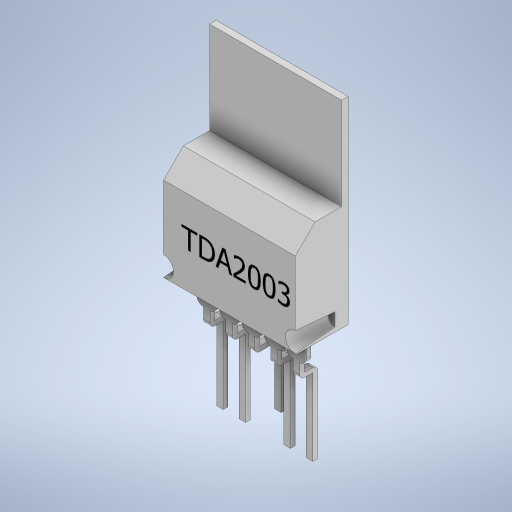
# Autodesk Inventor part: TDA2003
Saved by Autodesk Inventor 2024 (Build 280153000, 153)
## iProperties
Created: 2023-12-15
Part Number: TDA2003
Material: Generic
Document SubType Name: Sheet Metal
Designer: user
Density: 1 g/cm^3
Sheet Metal Rule: Default
Appearance: Default
Author: user
Autodesk Inventor part; units mm, degrees
sketch "Sketch1" plane through (0, 0, 0) normal (0, 0, 1) x (1, 0, 0)
  line L0 (0, 0) -> (10, 0)
  line L1 (10, 0) -> (10, 5)
  line L2 (10, 5) -> (0, 5)
  line L3 (0, 5) -> (0, 0)
  line L4 (0, 0) -> (0, 1.6)
  line L5 (0, 0) -> (0, 0.1)
  arc A0 (0, 0.1) -> (0, 1.6) centre (0, 0.85) ccw
  line L6 (10, 0) -> (10, 1.6)
  line L7 (10, 0) -> (10, 0.1)
  arc A1 (10, 1.6) -> (10, 0.1) centre (10, 0.85) ccw
  dimension "d0" = 10
  dimension "d1" = 5
  dimension "d2" = 1.6
  dimension "d3" = 0.1
  dimension "d4" = 0.75
  dimension "d5" = 1.6
  dimension "d6" = 0.1
  dimension "d7" = 0.75
  constraints: 16 end point, 4 point on circle, 4 point on line, 2 centre point, 2 parallel, 1 horizontal, 1 perpendicular
  measures "d0" distance of L2.end L1.end
  measures "d1" distance of L1.end L0.end
  measures "d2" distance of L0.start L4.end
  measures "d3" distance of L0.start L5.end
  measures "d4" radius of A0
  measures "d5" distance of L0.end L6.end
  measures "d6" distance of L0.end L7.end
  measures "d7" radius of A1
extrude "Extrusion1" add sketch "Sketch1" along normal blind 1 contours L3 A0 | A1 L1
extrude "Extrusion2" add sketch "Sketch1" along normal blind 4 contours L3 A0 L2 L1 A1 L0
draft "FaceDraft1" angle 5 pull direction (0, 0, 1) faces at (9.8797, 0.1097, 2) fixed edges at (9.25, 0.85, 4)
draft "FaceDraft2" angle 5 pull direction (0, 0, 1) faces at (0.0603, 0.1024, 3) fixed edges at (0.75, 0.85, 4)
sketch "Sketch2" plane through (0, 5, 0) normal (0, 1, 0) x (1, 0, 0)
  line L0 (0, -1) -> (0, -4) projected
  line L1 (10, 0) -> (0, 0) projected
  line L2 (0, -4) -> (10, -4)
  line L3 (10, -4) -> (10, 0)
  line L4 (10, 0) -> (0, 0)
  line L5 (0, 0) -> (0, -4)
  line L6 (0, 0) -> (10, 0)
  line L7 (10, 0) -> (10, -0.5)
  line L8 (10, -0.5) -> (0, -0.5)
  line L9 (0, -0.5) -> (0, 0)
  dimension "d14" = 0.5
  constraints: 16 end point, 4 parallel, 2 horizontal, 2 perpendicular, 1 point on line
  measures "d14" distance of L6.end L7.end
extrude "Extrusion3" add sketch "Sketch2" along normal blind 3
sketch "Sketch3" plane through (0, 8, 0) normal (0, 1, 0) x (1, 0, 0)
  line L0 (10, 0) -> (10, -4) projected
  line L1 (0, 0) -> (10, 0)
  line L2 (10, 0) -> (10, -0.5)
  line L3 (10, -0.5) -> (0, -0.5)
  line L4 (0, -0.5) -> (0, 0)
  dimension "d17" = 0.5
  constraints: 8 end point, 2 parallel, 1 horizontal, 1 perpendicular, 1 point on line
  measures "d17" distance of L1.end L2.end
extrude "Extrusion4" add sketch "Sketch3" along normal blind 7
chamfer "Chamfer1" distance 1.5 angle 45 1 edges at (5, 8, 4)
chamfer "Chamfer2" distance 0.1 angle 45 1 edges at (5, 0, 4)
sketch "Sketch4" plane through (0, 0, 0) normal (0, -1, 0) x (1, 0, 0)
  line L0 (0.75, 1.9689) -> (2.45, 1.9689)
  line L1 (2.45, 1.9689) -> (4.15, 1.9689)
  line L2 (4.15, 1.9689) -> (5.85, 1.9689)
  line L3 (5.85, 1.9689) -> (7.55, 1.9689)
  line L4 (7.55, 1.9689) -> (9.25, 1.9689)
  line L5 (10, 0) -> (10, 3.9) projected
  line L6 (0, 3.9) -> (10, 3.9) projected
  line L7 (3.3, 1.9689) -> (3.3, 3.9)
  line L8 (5, 1.9689) -> (5, 3.9)
  line L9 (6.7, 1.9689) -> (6.7, 3.9)
  line L10 (8.4, 1.9689) -> (8.4, 3.9)
  line L11 (0.75, 1.9689) -> (0.85, 1.9689)
  line L12 (2.45, 1.9689) -> (2.55, 1.9689)
  line L13 (4.15, 1.9689) -> (4.25, 1.9689)
  line L14 (5.85, 1.9689) -> (5.95, 1.9689)
  line L15 (7.55, 1.9689) -> (7.65, 1.9689)
  line L16 (0.85, 1.9689) -> (2.35, 1.9689)
  line L17 (2.35, 1.9689) -> (2.35, 2.3189)
  line L18 (2.35, 2.3189) -> (0.85, 2.3189)
  line L19 (0.85, 2.3189) -> (0.85, 1.9689)
  line L20 (2.55, 1.9689) -> (4.05, 1.9689)
  line L21 (4.05, 1.9689) -> (4.05, 2.3189)
  line L22 (4.05, 2.3189) -> (2.55, 2.3189)
  line L23 (2.55, 2.3189) -> (2.55, 1.9689)
  line L24 (4.25, 1.9689) -> (5.75, 1.9689)
  line L25 (5.75, 1.9689) -> (5.75, 2.3189)
  line L26 (5.75, 2.3189) -> (4.25, 2.3189)
  line L27 (4.25, 2.3189) -> (4.25, 1.9689)
  line L28 (5.95, 1.9689) -> (7.45, 1.9689)
  line L29 (7.45, 1.9689) -> (7.45, 2.3189)
  line L30 (7.45, 2.3189) -> (5.95, 2.3189)
  line L31 (5.95, 2.3189) -> (5.95, 1.9689)
  line L32 (7.65, 1.9689) -> (9.15, 1.9689)
  line L33 (9.15, 1.9689) -> (9.15, 2.3189)
  line L34 (9.15, 2.3189) -> (7.65, 2.3189)
  line L35 (7.65, 2.3189) -> (7.65, 1.9689)
  line L36 (1.6, 1.9689) -> (1.6, 3.9)
  point P0 (0, 0)
  dimension "d27" = 1.7
  dimension "d28" = 1.7
  dimension "d29" = 1.7
  dimension "d30" = 1.7
  dimension "d31" = 1.7
  dimension "d32" = 0.1
  dimension "d33" = 0.1
  dimension "d34" = 0.1
  dimension "d35" = 0.1
  dimension "d36" = 0.1
  dimension "d37" = 1.5
  dimension "d38" = 0.35
  dimension "d39" = 1.5
  dimension "d40" = 0.35
  dimension "d41" = 1.5
  dimension "d42" = 0.35
  dimension "d43" = 1.5
  dimension "d44" = 0.35
  dimension "d45" = 1.5
  dimension "d46" = 0.35
  constraints: 70 end point, 13 point on line, 10 parallel, 9 perpendicular, 6 midpoint, 5 horizontal
  measures "d27" distance of L0.start L0.end
  measures "d28" distance of L0.end L1.end
  measures "d29" distance of L1.end L2.end
  measures "d30" distance of L2.end L3.end
  measures "d31" distance of L3.end L4.end
  measures "d32" distance of L0.start L11.end
  measures "d33" distance of L0.end L12.end
  measures "d34" distance of L1.end L13.end
  measures "d35" distance of L2.end L14.end
  measures "d36" distance of L3.end L15.end
  measures "d37" distance of L18.end L17.end
  measures "d38" distance of L17.end L16.end
  measures "d39" distance of L22.end L21.end
  measures "d40" distance of L21.end L20.end
  measures "d41" distance of L26.end L25.end
  measures "d42" distance of L25.end L24.end
  measures "d43" distance of L30.end L29.end
  measures "d44" distance of L29.end L28.end
  measures "d45" distance of L34.end L33.end
  measures "d46" distance of L33.end L32.end
ref_plane "Work Plane2" through (3.3, 0, 1.9689) normal (1, 0, 0) x (0, 0, 1)
ref_plane "Work Plane3" through (5, 0, 1.9689) normal (1, 0, 0) x (0, 0, 1)
ref_plane "Work Plane4" through (6.7, 0, 1.9689) normal (1, 0, 0) x (0, 0, 1)
ref_plane "Work Plane5" through (8.4, 0, 1.9689) normal (1, 0, 0) x (0, 0, 1)
extrude "Extrusion5" add sketch "Sketch4" along normal blind 2 contours L19 L18 L36 L0 | L36 L18 L17 L0 | L23 L22 L7 L1 | L7 L22 L21 L1 | L26 L25 L2 L8 | L8 L2 L27 L26 | L30 L29 L3 L9 | L9 L3 L31 L30 | L34 L33 L4 L10 | L10 L4 L35 L34
fillet "Fillet1" radius 0.5 10 edges at (2.35, -2, 2.1439) (0.85, -2, 2.1439) (2.55, -2, 2.1439) (4.05, -2, 2.1439) (4.25, -2, 2.1439) (5.75, -2, 2.1439) (5.95, -2, 2.1439) (7.45, -2, 2.1439) (7.65, -2, 2.1439) (9.15, -2, 2.1439)
sketch "Sketch5" plane through (8.4, 0, 1.9689) normal (1, 0, 0) x (0, 0, 1)
  line L0 (0.1751, 0) -> (0.1751, 2)
  line L1 (0.1751, 2) -> (0.1751, 2.8)
  line L2 (-0.0249, 3) -> (-0.6249, 3)
  line L3 (-0.8249, 3.2) -> (-0.8249, 9)
  arc A0 (0.1751, 2.8) -> (-0.0249, 3) centre (-0.0249, 2.8) ccw
  arc A1 (-0.8249, 3.2) -> (-0.6249, 3) centre (-0.6249, 3.2) ccw
  point P0 (-1.9689, 0)
  point P1 (1.9311, 0)
  point P2 (0.1751, 3)
  point P3 (-0.8249, 3)
  dimension "d55" = 1.756
  dimension "d56" = 2
  dimension "d57" = 1
  dimension "d58" = 1
  dimension "d59" = 6
  dimension "d60" = 0.2
  constraints: 8 end point, 5 point on line, 4 point on circle, 4 tangent, 2 centre point, 2 perpendicular, 1 equal radius
  measures "d55" distance of point (1.931, 0) L0.start
  measures "d56" distance of L0.start L0.end
  measures "d57" distance of L0.end point (0.175, 3)
  measures "d58" distance of point (0.175, 3) point (-0.825, 3)
  measures "d59" distance of point (-0.825, 3) L3.end
  measures "d60" radius of A0
ref_plane "Work Plane6" through (0, -2, 0) normal (0, -1, 0) x (1, 0, 0)
ref_plane "Work Plane7" through (0, -2, 0) normal (0, -1, 0) x (1, 0, 0)
ref_plane "Work Plane8" through (0, -2, 0) normal (0, -1, 0) x (1, 0, 0)
ref_plane "Work Plane9" through (0, -2, 0) normal (0, -1, 0) x (1, 0, 0)
ref_plane "Work Plane10" through (0, -2, 0) normal (0, -1, 0) x (1, 0, 0)
sketch "Sketch6" plane through (0, -2, 0) normal (0, -1, 0) x (1, 0, 0)
  line L0 (8.65, 2.3189) -> (8.15, 2.3189) projected
  line L1 (8.15, 1.9689) -> (8.65, 1.9689) projected
  line L2 (8.65, 2.3189) -> (8.15, 2.3189)
  line L3 (8.15, 2.3189) -> (8.15, 1.9689)
  line L4 (8.15, 1.9689) -> (8.65, 1.9689)
  line L5 (8.65, 1.9689) -> (8.65, 2.3189)
  point P0 (0, 0)
  constraints: 8 end point, 2 parallel, 1 horizontal, 1 perpendicular
sketch "Sketch7" plane through (6.7, 0, 1.9689) normal (1, 0, 0) x (0, 0, 1)
  line L0 (0.1751, 0) -> (0.1751, 2)
  line L1 (0.1751, 2) -> (0.1751, 2.8)
  line L2 (-0.0249, 3) -> (-0.6249, 3)
  line L3 (-0.8249, 3.2) -> (-0.8249, 9)
  arc A0 (0.1751, 2.8) -> (-0.0249, 3) centre (-0.0249, 2.8) ccw
  arc A1 (-0.8249, 3.2) -> (-0.6249, 3) centre (-0.6249, 3.2) ccw
  point P0 (-1.9689, 0)
  point P1 (1.9311, 0)
  point P2 (0.1751, 3)
  point P3 (-0.8249, 3)
  dimension "d66" = 1.756
  dimension "d67" = 2
  dimension "d68" = 1
  dimension "d69" = 1
  dimension "d70" = 6
  dimension "d71" = 0.2
  constraints: 8 end point, 5 point on line, 4 point on circle, 4 tangent, 2 centre point, 2 perpendicular, 1 equal radius
  measures "d66" distance of point (1.931, 0) L0.start
  measures "d67" distance of L0.start L0.end
  measures "d68" distance of L0.end point (0.175, 3)
  measures "d69" distance of point (0.175, 3) point (-0.825, 3)
  measures "d70" distance of point (-0.825, 3) L3.end
  measures "d71" radius of A0
sketch "Sketch8" plane through (5, 0, 1.9689) normal (1, 0, 0) x (0, 0, 1)
  line L0 (0.1751, 0) -> (0.1751, 2)
  line L1 (0.1751, 2) -> (0.1751, 2.8)
  line L2 (-0.0249, 3) -> (-1.6249, 3)
  line L3 (-1.8249, 3.2) -> (-1.8249, 8)
  arc A0 (0.1751, 2.8) -> (-0.0249, 3) centre (-0.0249, 2.8) ccw
  arc A1 (-1.8249, 3.2) -> (-1.6249, 3) centre (-1.6249, 3.2) ccw
  point P0 (-1.9689, 0)
  point P1 (1.9311, 0)
  point P2 (-0.8249, 3)
  point P3 (0.1751, 3)
  point P4 (-1.8249, 3)
  dimension "d72" = 1.756
  dimension "d73" = 2
  dimension "d92" = 1
  dimension "d93" = 2
  dimension "d94" = 5
  dimension "d100" = 0.2
  constraints: 8 end point, 4 point on circle, 4 point on line, 4 tangent, 2 centre point, 2 perpendicular, 1 equal radius, 1 vertical
  measures "d72" distance of point (1.931, 0) L0.start
  measures "d73" distance of L0.start L0.end
  measures "d92" distance of L0.end point (0.175, 3)
  measures "d93" distance of point (0.175, 3) point (-1.825, 3)
  measures "d94" distance of point (-1.825, 3) L3.end
  measures "d100" radius of A0
sketch "Sketch9" plane through (3.3, 0, 1.9689) normal (1, 0, 0) x (0, 0, 1)
  line L0 (0.1751, 0) -> (0.1751, 2)
  line L1 (0.1751, 2) -> (0.1751, 2.8)
  line L2 (-0.0249, 3) -> (-0.6249, 3)
  line L3 (-0.8249, 3.2) -> (-0.8249, 9)
  arc A0 (0.1751, 2.8) -> (-0.0249, 3) centre (-0.0249, 2.8) ccw
  arc A1 (-0.8249, 3.2) -> (-0.6249, 3) centre (-0.6249, 3.2) ccw
  point P0 (-1.9689, 0)
  point P1 (1.9311, 0)
  point P2 (0.1751, 3)
  point P3 (-0.8249, 3)
  dimension "d78" = 1.756
  dimension "d79" = 2
  dimension "d80" = 1
  dimension "d81" = 1
  dimension "d82" = 6
  dimension "d83" = 0.2
  constraints: 8 end point, 5 point on line, 4 point on circle, 4 tangent, 2 centre point, 2 perpendicular, 1 equal radius
  measures "d78" distance of point (1.931, 0) L0.start
  measures "d79" distance of L0.start L0.end
  measures "d80" distance of L0.end point (0.175, 3)
  measures "d81" distance of point (0.175, 3) point (-0.825, 3)
  measures "d82" distance of point (-0.825, 3) L3.end
  measures "d83" radius of A0
ref_plane "Work Plane12" through (1.6, 0, 1.9689) normal (1, 0, 0) x (0, 0, 1)
sketch "Sketch10" plane through (1.6, 0, 1.9689) normal (1, 0, 0) x (0, 0, 1)
  line L0 (0.1751, 0) -> (0.1751, 2)
  line L1 (0.1751, 2) -> (0.1751, 2.8)
  line L2 (-0.0249, 3) -> (-0.6249, 3)
  line L3 (-0.8249, 3.2) -> (-0.8249, 9)
  arc A0 (0.1751, 2.8) -> (-0.0249, 3) centre (-0.0249, 2.8) ccw
  arc A1 (-0.8249, 3.2) -> (-0.6249, 3) centre (-0.6249, 3.2) ccw
  point P0 (-1.9689, 0)
  point P1 (1.9311, 0)
  point P2 (0.1751, 3)
  point P3 (-0.8249, 3)
  dimension "d86" = 1.756
  dimension "d87" = 2
  dimension "d88" = 1
  dimension "d89" = 1
  dimension "d90" = 6
  dimension "d91" = 0.2
  constraints: 8 end point, 5 point on line, 4 point on circle, 4 tangent, 2 centre point, 2 perpendicular, 1 equal radius
  measures "d86" distance of point (1.931, 0) L0.start
  measures "d87" distance of L0.start L0.end
  measures "d88" distance of L0.end point (0.175, 3)
  measures "d89" distance of point (0.175, 3) point (-0.825, 3)
  measures "d90" distance of point (-0.825, 3) L3.end
  measures "d91" radius of A0
sketch "Sketch14" plane through (0, -2, 0) normal (0, -1, 0) x (1, 0, 0)
  line L0 (6.95, 2.3189) -> (6.95, 1.9689) projected
  line L1 (7.45, 1.9689) -> (5.95, 1.9689) projected
  line L2 (6.95, 2.3189) -> (6.45, 2.3189)
  line L3 (6.45, 2.3189) -> (6.45, 1.9689)
  line L4 (6.45, 1.9689) -> (6.95, 1.9689)
  line L5 (6.95, 1.9689) -> (6.95, 2.3189)
  point P0 (0, 0)
  dimension "d95" = 0.5
  constraints: 8 end point, 2 parallel, 1 horizontal, 1 perpendicular, 1 point on line
  measures "d95" distance of L4.end L3.end
sketch "Sketch15" plane through (0, -2, 0) normal (0, -1, 0) x (1, 0, 0)
  line L0 (5.25, 2.3189) -> (5.25, 1.9689) projected
  line L1 (4.25, 2.3189) -> (5.75, 2.3189) projected
  line L2 (5.25, 1.9689) -> (4.7503, 1.9689)
  line L3 (4.7503, 1.9689) -> (4.7503, 2.3189)
  line L4 (4.7503, 2.3189) -> (5.25, 2.3189)
  line L5 (5.25, 2.3189) -> (5.25, 1.9689)
  point P0 (0, 0)
  constraints: 8 end point, 2 parallel, 1 horizontal, 1 perpendicular, 1 point on line
sketch "Sketch16" plane through (0, -2, 0) normal (0, -1, 0) x (1, 0, 0)
  line L0 (3.05, 1.9689) -> (3.05, 2.3189) projected
  line L1 (4.05, 1.9689) -> (2.55, 1.9689) projected
  line L2 (3.05, 2.3189) -> (3.5503, 2.3189)
  line L3 (3.5503, 2.3189) -> (3.5503, 1.9689)
  line L4 (3.5503, 1.9689) -> (3.05, 1.9689)
  line L5 (3.05, 1.9689) -> (3.05, 2.3189)
  point P0 (0, 0)
  constraints: 8 end point, 2 parallel, 1 horizontal, 1 perpendicular, 1 point on line
sketch "Sketch17" plane through (0, -2, 0) normal (0, -1, 0) x (1, 0, 0)
  line L0 (1.85, 2.3189) -> (1.85, 1.9689) projected
  line L1 (2.35, 1.9689) -> (0.85, 1.9689) projected
  line L2 (1.85, 2.3189) -> (1.35, 2.3189)
  line L3 (1.35, 2.3189) -> (1.35, 1.9689)
  line L4 (1.35, 1.9689) -> (1.85, 1.9689)
  line L5 (1.85, 1.9689) -> (1.85, 2.3189)
  point P0 (0, 0)
  constraints: 8 end point, 2 parallel, 1 horizontal, 1 perpendicular, 1 point on line
sweep "Sweep1" add profiles "Sketch14" path "Sketch7"
sweep "Sweep2" add profiles "Sketch6" path "Sketch5"
sweep "Sweep3" add profiles "Sketch15" path "Sketch8"
sweep "Sweep4" add profiles "Sketch16" path "Sketch9"
sweep "Sweep5" add profiles "Sketch17" path "Sketch10"
sketch "Sketch18" plane through (0, 0, 4) normal (0, 0, 1) x (1, 0, 0)
  line L0 (1.3584, 4.3277) -> (18.3126, 4.3277) construction
  line L1 (18.3126, 4.3277) -> (18.3126, 1.1513) construction
  line L2 (18.3126, 1.1513) -> (1.3584, 1.1513) construction
  line L3 (1.3584, 1.1513) -> (1.3584, 4.3277) construction
  point P0 (0, 0)
  constraints: 2 other
equation "\"BendRadius\" = Thickness"
equation "\"BendReliefWidth\" = Thickness"
equation "\"BendReliefDepth\" = 0.5 * Thickness"
equation "\"CornerReliefSize\" = 4 * Thickness"
equation "\"MinimumRemnant\" = 2 * Thickness"
equation "\"TransitionRadius\" = BendRadius"
equation "\"JacobiRadiusSize\" = BendRadius"
equation "\"GapSize\" = Thickness"
equation "\"Thickness\" = 3.048"
body "Solid1"
